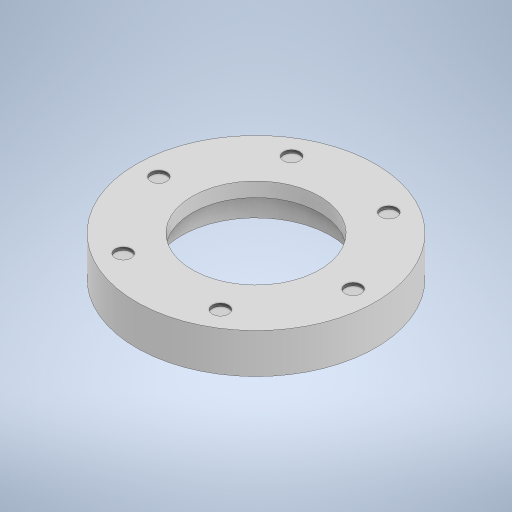
# Autodesk Inventor part: 9_AnilloComplementarioA
Saved by Autodesk Inventor 2024.2 (Build 282272000, 272)
## iProperties
Created: 2024-04-26
Part Number: 9_AnilloComplementarioA
Material: Genérico
Document SubType Name: Modeling
Designer: Cosmic Dinodog
Density: 1 g/cm^3
Appearance: Valor por defecto
Author: Cosmic Dinodog
Autodesk Inventor part; units mm, degrees
ref_plane "YZ Plane" through (0, 0, 0) normal (1, 0, 0) x (0, 1, 0)
ref_plane "XZ Plane" through (0, 0, 0) normal (0, 1, 0) x (-1, 0, 0)
ref_plane "XY Plane" through (0, 0, 0) normal (0, 0, 1) x (1, 0, 0)
sketch "Boceto1" plane through (0, 0, 0) normal (0, 1, 0) x (-1, 0, 0)
  circle A0 centre (0, 0) radius 75
  circle A1 centre (0, 0) radius 40
  dimension "d0" = 150
  dimension "d1" = 80
  constraints: 2 centre point, 2 coincident
  measures "d0" diameter of A0
  measures "d1" diameter of A1
extrude "Extrusión1" add sketch "Boceto1" along normal blind 25
sketch "Boceto2" plane through (0, 0, 0) normal (0, -1, 0) x (1, 0, 0)
  circle A0 centre (0, 0) radius 47
  dimension "d4" = 94
  constraints: 1 centre point, 1 coincident
  measures "d4" diameter of A0
extrude "Extrusión2" cut sketch "Boceto2" against normal blind 16
sketch "Boceto3" plane through (0, 25, 0) normal (0, 1, 0) x (1, 0, 0)
  circle A0 centre (0, 0) radius 61
  line L0 (0, 0) -> (61, 0) construction
  point P0 (30.5, 52.8275)
  point P1 (-30.5, 52.8275)
  point P2 (-61, 0)
  point P3 (-30.5, -52.8275)
  point P4 (30.5, -52.8275)
  dimension "d7" = 122
  dimension "d10" = 360
  constraints: 2 coincident, 2 end point, 1 horizontal, 1 horizontal alignment, 9 other
hole "Agujero1" at (61, 25, 0) at (30.5, 25, -52.8275) at (-30.5, 25, -52.8275) at (-61, 25, 0) at (-30.5, 25, 52.8275) at (30.5, 25, 52.8275) direction (0, -1, 0) diameter 10.106 depth 1.75 thread size "M12x1.75" class "6H" standard "ISO Metric profile"
